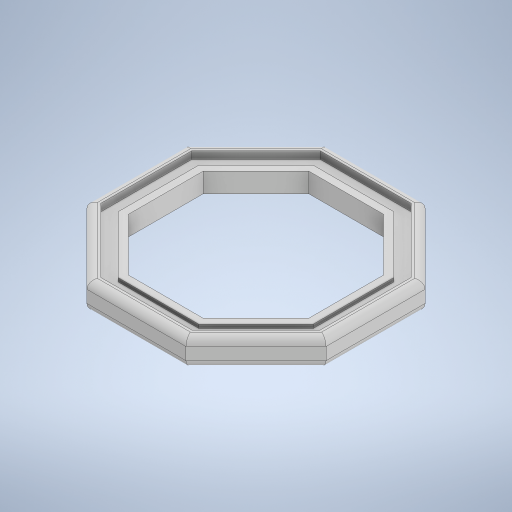
# Autodesk Inventor part: OV-PAM_ring_2
Saved by Autodesk Inventor 2024 (Build 280153000, 153)
## iProperties
Created: 2023-06-19
Part Number: OV-PAM_ring_2
Material: 일반
Document SubType Name: Modeling
Designer: jsw
Density: 1 g/cm^3
Appearance: 기본값
Author: jsw
Autodesk Inventor part; units mm, degrees
ref_plane "YZ Plane" through (0, 0, 0) normal (1, 0, 0) x (0, 1, 0)
ref_plane "XZ Plane" through (0, 0, 0) normal (0, 1, 0) x (-1, 0, 0)
sketch "스케치1" plane through (0, 0, 0) normal (0, 1, 0) x (-1, 0, 0)
  line L0 (-16.2959, 6.75) -> (-6.75, 16.2959)
  line L1 (-6.75, 16.2959) -> (6.75, 16.2959)
  line L2 (6.75, 16.2959) -> (16.2959, 6.75)
  line L3 (16.2959, 6.75) -> (16.2959, -6.75)
  line L4 (16.2959, -6.75) -> (6.75, -16.2959)
  line L5 (6.75, -16.2959) -> (-6.75, -16.2959)
  line L6 (-6.75, -16.2959) -> (-16.2959, -6.75)
  line L7 (-16.2959, -6.75) -> (-16.2959, 6.75)
  line L8 (19.4959, 8.0755) -> (19.4959, -8.0755)
  line L9 (19.4959, -8.0755) -> (8.0755, -19.4959)
  line L10 (8.0755, -19.4959) -> (-8.0755, -19.4959)
  line L11 (-8.0755, -19.4959) -> (-19.4959, -8.0755)
  line L12 (-19.4959, -8.0755) -> (-19.4959, 8.0755)
  line L13 (-19.4959, 8.0755) -> (-8.0755, 19.4959)
  line L14 (-8.0755, 19.4959) -> (8.0755, 19.4959)
  line L15 (8.0755, 19.4959) -> (19.4959, 8.0755)
  point P0 (0, 0)
  point P1 (0, 0)
  point P2 (0, 0)
  dimension "d0" = 13.5
  dimension "d1" = 3.2
  constraints: 32 end point, 2 coincident, 2 horizontal, 34 other
  measures "d0" distance of L2.end L3.end
  measures "d1" distance between parallel lines of L8 L3
extrude "돌출1" add sketch "스케치1" along normal blind 4.4 contours L0 L1 L2 L3 L4 L5 L6 L7 | L8 L9 L10 L11 L12 L13 L14 L15
sketch "스케치14" plane through (0, 4.4, 0) normal (0, 1, 0) x (1, 0, 0)
  line L0 (6.5843, -15.8959) -> (-6.5843, -15.8959)
  line L1 (-6.5843, -15.8959) -> (-15.8959, -6.5843)
  line L2 (-15.8959, -6.5843) -> (-15.8959, 6.5843)
  line L3 (-15.8959, 6.5843) -> (-6.5843, 15.8959)
  line L4 (-6.5843, 15.8959) -> (6.5843, 15.8959)
  line L5 (6.5843, 15.8959) -> (15.8959, 6.5843)
  line L6 (15.8959, 6.5843) -> (15.8959, -6.5843)
  line L7 (15.8959, -6.5843) -> (6.5843, -15.8959)
  line L8 (-7.4127, 17.8959) -> (7.4127, 17.8959)
  line L9 (7.4127, 17.8959) -> (17.8959, 7.4127)
  line L10 (17.8959, 7.4127) -> (17.8959, -7.4127)
  line L11 (17.8959, -7.4127) -> (7.4127, -17.8959)
  line L12 (7.4127, -17.8959) -> (-7.4127, -17.8959)
  line L13 (-7.4127, -17.8959) -> (-17.8959, -7.4127)
  line L14 (-17.8959, -7.4127) -> (-17.8959, 7.4127)
  line L15 (-17.8959, 7.4127) -> (-7.4127, 17.8959)
  line L16 (19.4959, -8.0755) -> (19.4959, 8.0755) projected
  point P0 (0, 0)
  point P1 (0, 0)
  point P2 (0, 0)
  dimension "d138" = 2
  dimension "d139" = 1.6
  constraints: 32 end point, 2 coincident, 2 horizontal, 34 other
  measures "d138" distance between parallel lines of L10 L6
  measures "d139" distance between parallel lines of L10 L16
extrude "돌출16" cut sketch "스케치14" against normal blind 1.2
sketch "스케치15" plane through (0, 4.4, 0) normal (0, 1, 0) x (1, 0, 0)
  line L0 (-15.8959, -6.5843) -> (-6.5843, -15.8959) projected
  line L1 (-6.5843, -15.8959) -> (6.5843, -15.8959) projected
  line L2 (6.5843, -15.8959) -> (15.8959, -6.5843) projected
  line L3 (15.8959, -6.5843) -> (15.8959, 6.5843) projected
  line L4 (15.8959, 6.5843) -> (6.5843, 15.8959) projected
  line L5 (6.5843, 15.8959) -> (-6.5843, 15.8959) projected
  line L6 (-6.5843, 15.8959) -> (-15.8959, 6.5843) projected
  line L7 (-15.8959, 6.5843) -> (-15.8959, -6.5843) projected
  point P0 (0, 0)
extrude "돌출17" cut sketch "스케치15" against normal blind 0.6
sketch "스케치16" plane through (0, 3.8, 0) normal (0, 1, 0) x (1, 0, 0)
  line L0 (-6.0873, 14.6959) -> (6.0873, 14.6959)
  line L1 (6.0873, 14.6959) -> (14.6959, 6.0873)
  line L2 (14.6959, 6.0873) -> (14.6959, -6.0873)
  line L3 (14.6959, -6.0873) -> (6.0873, -14.6959)
  line L4 (6.0873, -14.6959) -> (-6.0873, -14.6959)
  line L5 (-6.0873, -14.6959) -> (-14.6959, -6.0873)
  line L6 (-14.6959, -6.0873) -> (-14.6959, 6.0873)
  line L7 (-14.6959, 6.0873) -> (-6.0873, 14.6959)
  line L8 (15.8959, 6.5843) -> (15.8959, -6.5843) projected
  point P0 (0, 0)
  point P1 (0, 0)
  dimension "d144" = 1.2
  constraints: 16 end point, 1 coincident, 1 horizontal, 17 other
  measures "d144" distance between parallel lines of L2 L8
extrude "돌출18" cut sketch "스케치16" against normal up to surface (3.8 mm away)
fillet "모깎기2" radius 1.2 16 edges at (0, 4.4, -19.4959) (-13.7857, 4.4, -13.7857) (13.7857, 4.4, -13.7857) (19.4959, 4.4, 0) (13.7857, 4.4, 13.7857) (0, 4.4, 19.4959) (-13.7857, 4.4, 13.7857) (-19.4959, 4.4, 0) (-19.4959, 0, 0) (-13.7857, 0, 13.7857) (0, 0, 19.4959) (13.7857, 0, 13.7857) (-13.7857, 0, -13.7857) (0, 0, -19.4959) (19.4959, 0, 0) (13.7857, 0, -13.7857)
ref_plane "작업 평면3" through (0, 2.2, 0) normal (0, -1, 0) x (1, 0, 0)
mirror "미러6" about plane through (0, 2.2, 0) normal (0, -1, 0) of "돌출17", "돌출16"
